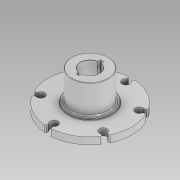
# Autodesk Inventor part: am-0976
Saved by Autodesk Inventor 2020.1 (Build 241239000, 239)
## iProperties
Category: FIRSTChoice
Company: Autodesk Inc.
Created: 2019-11-26
Part Number: am-0976
Material: Aluminum 6061
Document SubType Name: Modeling
Designer: Autodesk Inc.
Density: 2.7 g/cm^3
Appearance: Aluminum - Polished
Catalog Web Link: https://www.andymark.com/products/500ex-key-hub
Vendor: AndyMark Inc.
Author: Autodesk Inc.
Autodesk Inventor part; units mm, degrees
ref_plane "YZ Plane" through (0, 0, 0) normal (1, 0, 0) x (0, 1, 0)
ref_plane "XZ Plane" through (0, 0, 0) normal (0, 1, 0) x (-1, 0, 0)
sketch "Sketch1" plane through (0, 0, 0) normal (0, 1, 0) x (-1, 0, 0)
  circle A0 centre (0, 0) radius 27.7876
  circle A1 centre (0, 0) radius 23.8125 construction
  line L0 (0, 0) -> (28.7391, -16.5925) construction
  line L1 (0, 0) -> (27.7876, 0) construction
  dimension "d0" = 55.5752
  dimension "d1" = 47.625
  dimension "d2" = 30
  constraints: 4 end point, 2 coincident, 1 centre point, 1 horizontal, 1 horizontal alignment, 2 other
  measures "d1" diameter of A1
  measures "d2" angle of L1 L0
extrude "Extrusion1" add sketch "Sketch1" against normal blind 4.572
sketch "Sketch2" plane through (0, 0, 0) normal (0, 1, 0) x (1, 0, 0)
  circle A0 centre (0, 0) radius 23.8125 construction
  line L0 (0, 0) -> (-24.0648, 13.8938) construction
  circle A1 centre (0, 0) radius 27.7876 construction
  line L1 (0, 0) -> (27.7876, 0) construction
  point P0 (-20.6222, 11.9062)
  dimension "d5" = 47.625
  dimension "d6" = 150
  constraints: 4 end point, 1 coincident, 1 equal length, 1 horizontal, 1 point on line, 5 other
  measures "d6" angle of L1 L0
hole "Hole1" at (-20.6222, 0, -11.9062) direction (0, -1, 0) diameter 5.1816 end through all
sketch "Sketch3" plane through (0, 0, 0) normal (0, 1, 0) x (1, 0, 0)
  circle A0 centre (-20.6222, 11.9062) radius 2.5908 projected
  line L0 (0, 0) -> (-20.6222, 11.9062) construction
  line L1 (-23.1891, 11.5552) -> (-24.8192, 12.4963)
  line L2 (-21.6016, 14.3048) -> (-23.2317, 15.2459)
  circle A1 centre (0, 0) radius 27.7876 projected
  dimension "d14" = 3.175
  dimension "d15" = 1.5875
  constraints: 6 end point, 4 point on circle, 2 parallel
  measures "d14" distance between parallel lines of L2 L1
  measures "d15" distance from line of L0.end L1
extrude "Extrusion2" cut sketch "Sketch3" against normal blind 7.9375 contours A0 L1 A1 L2 picked at (-23.1856, 14.4185)
fillet "Fillet1" radius 0.762 4 edges at (-23.1891, -2.286, -11.5552) (-24.8192, -2.286, -12.4963) (-21.6016, -2.286, -14.3048) (-23.2317, -2.286, -15.2459)
pattern_circular "Circular Pattern1" count 6 over 360 about axis through (0, 0, 0) along (0, -1, 0) of "Hole1", "Extrusion2", "Fillet1"
sketch "Sketch4" plane through (0, 0, 0) normal (0, 1, 0) x (1, 0, 0)
  circle A0 centre (0, 0) radius 14.2875
  dimension "d22" = 28.575
  constraints: 1 centre point, 1 coincident
  measures "d22" diameter of A0
extrude "Extrusion3" add sketch "Sketch4" along normal blind 0.889
chamfer "Chamfer1" distance 0.254 angle 45 1 edges at (-14.2875, 0.889, 0)
fillet "Fillet2" radius 0.254 1 edges at (-14.2875, 0, 0)
ref_plane "Work Plane1" through (0, -2.286, 0) normal (0, 1, 0) x (1, 0, 0)
mirror "Mirror1" about plane through (0, -2.286, 0) normal (0, 1, 0) of "Extrusion3"
chamfer "Chamfer2" distance 0.254 angle 45 1 edges at (-14.2875, -5.461, 0)
fillet "Fillet3" radius 0.254 1 edges at (-14.2875, -4.572, 0)
sketch "Sketch5" plane through (0, 0.889, 0) normal (0, 1, 0) x (1, 0, 0)
  circle A0 centre (0, 0) radius 12.192
  dimension "d33" = 24.384
  constraints: 1 centre point, 1 coincident
  measures "d33" diameter of A0
extrude "Extrusion4" add sketch "Sketch5" along normal blind 19.05
chamfer "Chamfer3" distance 0.254 angle 45 1 edges at (-12.192, 19.939, 0)
chamfer "Chamfer4" distance 0.8128 angle 45 1 edges at (-12.192, 0.889, 0)
sketch "Sketch6" plane through (0, 19.939, 0) normal (0, 1, 0) x (1, 0, 0)
  point P0 (0, 0)
hole "Hole2" at (0, 19.939, 0) direction (0, -1, 0) diameter 12.7 end through all
sketch "Sketch7" plane through (0, 19.939, 0) normal (0, 1, 0) x (1, 0, 0)
  line L0 (-1.1213, 6.2502) -> (-1.1213, 8.001)
  line L1 (1.1375, 6.2473) -> (1.1375, 8.001)
  line L2 (-1.1213, 8.001) -> (1.1375, 8.001)
  circle A0 centre (0, 0) radius 6.35 projected
  dimension "d49" = 8.001
  constraints: 6 end point, 2 point on circle, 2 vertical, 1 horizontal, 1 parallel
  measures "d49" distance from line of L2 point (0, 0)
extrude "Extrusion5" cut sketch "Sketch7" against normal through all contours L0 L2 L1 A0
mirror "Mirror2" about plane through (0, 0, 0) normal (0, 0, 1) of "Extrusion5"
fillet "Fillet4" radius 0.127 4 edges at (-1.1213, 7.239, -8.001) (1.1375, 7.239, -8.001) (-1.1213, 7.239, 8.001) (1.1375, 7.239, 8.001)
fillet "Fillet5" radius 0.127 2 edges at (-6.35, 19.939, 0) (6.35, 19.939, 0)
equation "\"d15\" = 0.5 * d14"
body "Solid1"
